Autodesk Inventor part; units mm, degrees
(part 2 of 2)
  arc A261 (1763.513924, 763.538309) -> (1755.513924, 771.538309) centre (1755.513924, 763.538309) ccw
  arc A262 (1755.513924, 731.538309) -> (1763.513924, 739.538309) centre (1755.513924, 739.538309) ccw
  arc A263 (1723.513924, 739.538309) -> (1731.513924, 731.538309) centre (1731.513924, 739.538309) ccw
  line L266 (2481.513924, 771.538309) -> (2505.513924, 771.538309)
  line L267 (2513.513924, 763.538309) -> (2513.513924, 739.538309)
  line L268 (2505.513924, 731.538309) -> (2481.513924, 731.538309)
  line L269 (2473.513924, 739.538309) -> (2473.513924, 763.538309)
  arc A264 (2481.513924, 771.538309) -> (2473.513924, 763.538309) centre (2481.513924, 763.538309) ccw
  arc A265 (2513.513924, 763.538309) -> (2505.513924, 771.538309) centre (2505.513924, 763.538309) ccw
  arc A266 (2505.513924, 731.538309) -> (2513.513924, 739.538309) centre (2505.513924, 739.538309) ccw
  arc A267 (2473.513924, 739.538309) -> (2481.513924, 731.538309) centre (2481.513924, 739.538309) ccw
  line L270 (3231.513924, 771.538309) -> (3255.513924, 771.538309)
  line L271 (3263.513924, 763.538309) -> (3263.513924, 739.538309)
  line L272 (3255.513924, 731.538309) -> (3231.513924, 731.538309)
  line L273 (3223.513924, 739.538309) -> (3223.513924, 763.538309)
  arc A268 (3231.513924, 771.538309) -> (3223.513924, 763.538309) centre (3231.513924, 763.538309) ccw
  arc A269 (3263.513924, 763.538309) -> (3255.513924, 771.538309) centre (3255.513924, 763.538309) ccw
  arc A270 (3255.513924, 731.538309) -> (3263.513924, 739.538309) centre (3255.513924, 739.538309) ccw
  arc A271 (3223.513924, 739.538309) -> (3231.513924, 731.538309) centre (3231.513924, 739.538309) ccw
  line L274 (3981.513924, 771.538309) -> (4005.513924, 771.538309)
  line L275 (4013.513924, 763.538309) -> (4013.513924, 739.538309)
  line L276 (4005.513924, 731.538309) -> (3981.513924, 731.538309)
  line L277 (3973.513924, 739.538309) -> (3973.513924, 763.538309)
  arc A272 (3981.513924, 771.538309) -> (3973.513924, 763.538309) centre (3981.513924, 763.538309) ccw
  arc A273 (4013.513924, 763.538309) -> (4005.513924, 771.538309) centre (4005.513924, 763.538309) ccw
  arc A274 (4005.513924, 731.538309) -> (4013.513924, 739.538309) centre (4005.513924, 739.538309) ccw
  arc A275 (3973.513924, 739.538309) -> (3981.513924, 731.538309) centre (3981.513924, 739.538309) ccw
  line L278 (4731.513924, 771.538309) -> (4755.513924, 771.538309)
  line L279 (4763.513924, 763.538309) -> (4763.513924, 739.538309)
  line L280 (4755.513924, 731.538309) -> (4731.513924, 731.538309)
  line L281 (4723.513924, 739.538309) -> (4723.513924, 763.538309)
  arc A276 (4731.513924, 771.538309) -> (4723.513924, 763.538309) centre (4731.513924, 763.538309) ccw
  arc A277 (4763.513924, 763.538309) -> (4755.513924, 771.538309) centre (4755.513924, 763.538309) ccw
  arc A278 (4755.513924, 731.538309) -> (4763.513924, 739.538309) centre (4755.513924, 739.538309) ccw
  arc A279 (4723.513924, 739.538309) -> (4731.513924, 731.538309) centre (4731.513924, 739.538309) ccw
  line L282 (231.513924, 21.538309) -> (255.513924, 21.538309)
  line L283 (263.513924, 13.538309) -> (263.513924, -10.461691)
  line L284 (255.513924, -18.461691) -> (231.513924, -18.461691)
  line L285 (223.513924, -10.461691) -> (223.513924, 13.538309)
  arc A280 (231.513924, 21.538309) -> (223.513924, 13.538309) centre (231.513924, 13.538309) ccw
  arc A281 (263.513924, 13.538309) -> (255.513924, 21.538309) centre (255.513924, 13.538309) ccw
  arc A282 (255.513924, -18.461691) -> (263.513924, -10.461691) centre (255.513924, -10.461691) ccw
  arc A283 (223.513924, -10.461691) -> (231.513924, -18.461691) centre (231.513924, -10.461691) ccw
  line L286 (981.513924, 21.538309) -> (1005.513924, 21.538309)
  line L287 (1013.513924, 13.538309) -> (1013.513924, -10.461691)
  line L288 (1005.513924, -18.461691) -> (981.513924, -18.461691)
  line L289 (973.513924, -10.461691) -> (973.513924, 13.538309)
  arc A284 (981.513924, 21.538309) -> (973.513924, 13.538309) centre (981.513924, 13.538309) ccw
  arc A285 (1013.513924, 13.538309) -> (1005.513924, 21.538309) centre (1005.513924, 13.538309) ccw
  arc A286 (1005.513924, -18.461691) -> (1013.513924, -10.461691) centre (1005.513924, -10.461691) ccw
  arc A287 (973.513924, -10.461691) -> (981.513924, -18.461691) centre (981.513924, -10.461691) ccw
  line L290 (1731.513924, 21.538309) -> (1755.513924, 21.538309)
  line L291 (1763.513924, 13.538309) -> (1763.513924, -10.461691)
  line L292 (1755.513924, -18.461691) -> (1731.513924, -18.461691)
  line L293 (1723.513924, -10.461691) -> (1723.513924, 13.538309)
  arc A288 (1731.513924, 21.538309) -> (1723.513924, 13.538309) centre (1731.513924, 13.538309) ccw
  arc A289 (1763.513924, 13.538309) -> (1755.513924, 21.538309) centre (1755.513924, 13.538309) ccw
  arc A290 (1755.513924, -18.461691) -> (1763.513924, -10.461691) centre (1755.513924, -10.461691) ccw
  arc A291 (1723.513924, -10.461691) -> (1731.513924, -18.461691) centre (1731.513924, -10.461691) ccw
  line L294 (2481.513924, 21.538309) -> (2505.513924, 21.538309)
  line L295 (2513.513924, 13.538309) -> (2513.513924, -10.461691)
  line L296 (2505.513924, -18.461691) -> (2481.513924, -18.461691)
  line L297 (2473.513924, -10.461691) -> (2473.513924, 13.538309)
  arc A292 (2481.513924, 21.538309) -> (2473.513924, 13.538309) centre (2481.513924, 13.538309) ccw
  arc A293 (2513.513924, 13.538309) -> (2505.513924, 21.538309) centre (2505.513924, 13.538309) ccw
  arc A294 (2505.513924, -18.461691) -> (2513.513924, -10.461691) centre (2505.513924, -10.461691) ccw
  arc A295 (2473.513924, -10.461691) -> (2481.513924, -18.461691) centre (2481.513924, -10.461691) ccw
  line L298 (3231.513924, 21.538309) -> (3255.513924, 21.538309)
  line L299 (3263.513924, 13.538309) -> (3263.513924, -10.461691)
  line L300 (3255.513924, -18.461691) -> (3231.513924, -18.461691)
  line L301 (3223.513924, -10.461691) -> (3223.513924, 13.538309)
  arc A296 (3231.513924, 21.538309) -> (3223.513924, 13.538309) centre (3231.513924, 13.538309) ccw
  arc A297 (3263.513924, 13.538309) -> (3255.513924, 21.538309) centre (3255.513924, 13.538309) ccw
  arc A298 (3255.513924, -18.461691) -> (3263.513924, -10.461691) centre (3255.513924, -10.461691) ccw
  arc A299 (3223.513924, -10.461691) -> (3231.513924, -18.461691) centre (3231.513924, -10.461691) ccw
  line L302 (3981.513924, 21.538309) -> (4005.513924, 21.538309)
  line L303 (4013.513924, 13.538309) -> (4013.513924, -10.461691)
  line L304 (4005.513924, -18.461691) -> (3981.513924, -18.461691)
  line L305 (3973.513924, -10.461691) -> (3973.513924, 13.538309)
  arc A300 (3981.513924, 21.538309) -> (3973.513924, 13.538309) centre (3981.513924, 13.538309) ccw
  arc A301 (4013.513924, 13.538309) -> (4005.513924, 21.538309) centre (4005.513924, 13.538309) ccw
  arc A302 (4005.513924, -18.461691) -> (4013.513924, -10.461691) centre (4005.513924, -10.461691) ccw
  arc A303 (3973.513924, -10.461691) -> (3981.513924, -18.461691) centre (3981.513924, -10.461691) ccw
  line L306 (4731.513924, 21.538309) -> (4755.513924, 21.538309)
  line L307 (4763.513924, 13.538309) -> (4763.513924, -10.461691)
  line L308 (4755.513924, -18.461691) -> (4731.513924, -18.461691)
  line L309 (4723.513924, -10.461691) -> (4723.513924, 13.538309)
  arc A304 (4731.513924, 21.538309) -> (4723.513924, 13.538309) centre (4731.513924, 13.538309) ccw
  arc A305 (4763.513924, 13.538309) -> (4755.513924, 21.538309) centre (4755.513924, 13.538309) ccw
  arc A306 (4755.513924, -18.461691) -> (4763.513924, -10.461691) centre (4755.513924, -10.461691) ccw
  arc A307 (4723.513924, -10.461691) -> (4731.513924, -18.461691) centre (4731.513924, -10.461691) ccw
  point P0 (0, 0)
  point P1 (263.513924, 7481.538309)
  point P2 (263.513924, 7521.538309)
  point P3 (223.513924, 7481.538309)
  point P4 (1013.513924, 7481.538309)
  point P5 (1013.513924, 7521.538309)
  point P6 (973.513924, 7481.538309)
  point P7 (1763.513924, 7481.538309)
  point P8 (1763.513924, 7521.538309)
  point P9 (1723.513924, 7481.538309)
  point P10 (2513.513924, 7481.538309)
  point P11 (2513.513924, 7521.538309)
  point P12 (2473.513924, 7481.538309)
  point P13 (3263.513924, 7481.538309)
  point P14 (3263.513924, 7521.538309)
  point P15 (3223.513924, 7481.538309)
  point P16 (4013.513924, 7481.538309)
  point P17 (4013.513924, 7521.538309)
  point P18 (3973.513924, 7481.538309)
  point P19 (4763.513924, 7481.538309)
  point P20 (4763.513924, 7521.538309)
  point P21 (4723.513924, 7481.538309)
  point P22 (263.513924, 6731.538309)
  point P23 (263.513924, 6771.538309)
  point P24 (223.513924, 6731.538309)
  point P25 (1013.513924, 6731.538309)
  point P26 (1013.513924, 6771.538309)
  point P27 (973.513924, 6731.538309)
  point P28 (1763.513924, 6731.538309)
  point P29 (1763.513924, 6771.538309)
  point P30 (1723.513924, 6731.538309)
  point P31 (2513.513924, 6731.538309)
  point P32 (2513.513924, 6771.538309)
  point P33 (2473.513924, 6731.538309)
  point P34 (3263.513924, 6731.538309)
  point P35 (3263.513924, 6771.538309)
  point P36 (3223.513924, 6731.538309)
  point P37 (4013.513924, 6731.538309)
  point P38 (4013.513924, 6771.538309)
  point P39 (3973.513924, 6731.538309)
  point P40 (4763.513924, 6731.538309)
  point P41 (4763.513924, 6771.538309)
  point P42 (4723.513924, 6731.538309)
  point P43 (263.513924, 5981.538309)
  point P44 (263.513924, 6021.538309)
  point P45 (223.513924, 5981.538309)
  point P46 (1013.513924, 5981.538309)
  point P47 (1013.513924, 6021.538309)
  point P48 (973.513924, 5981.538309)
  point P49 (1763.513924, 5981.538309)
  point P50 (1763.513924, 6021.538309)
  point P51 (1723.513924, 5981.538309)
  point P52 (2513.513924, 5981.538309)
  point P53 (2513.513924, 6021.538309)
  point P54 (2473.513924, 5981.538309)
  point P55 (3263.513924, 5981.538309)
  point P56 (3263.513924, 6021.538309)
  point P57 (3223.513924, 5981.538309)
  point P58 (4013.513924, 5981.538309)
  point P59 (4013.513924, 6021.538309)
  point P60 (3973.513924, 5981.538309)
  point P61 (4763.513924, 5981.538309)
  point P62 (4763.513924, 6021.538309)
  point P63 (4723.513924, 5981.538309)
  point P64 (263.513924, 5231.538309)
  point P65 (263.513924, 5271.538309)
  point P66 (223.513924, 5231.538309)
  point P67 (1013.513924, 5231.538309)
  point P68 (1013.513924, 5271.538309)
  point P69 (973.513924, 5231.538309)
  point P70 (1763.513924, 5231.538309)
  point P71 (1763.513924, 5271.538309)
  point P72 (1723.513924, 5231.538309)
  point P73 (2513.513924, 5231.538309)
  point P74 (2513.513924, 5271.538309)
  point P75 (2473.513924, 5231.538309)
  point P76 (3263.513924, 5231.538309)
  point P77 (3263.513924, 5271.538309)
  point P78 (3223.513924, 5231.538309)
  point P79 (4013.513924, 5231.538309)
  point P80 (4013.513924, 5271.538309)
  point P81 (3973.513924, 5231.538309)
  point P82 (4763.513924, 5231.538309)
  point P83 (4763.513924, 5271.538309)
  point P84 (4723.513924, 5231.538309)
  point P85 (263.513924, 4481.538309)
  point P86 (263.513924, 4521.538309)
  point P87 (223.513924, 4481.538309)
  point P88 (1013.513924, 4481.538309)
  point P89 (1013.513924, 4521.538309)
  point P90 (973.513924, 4481.538309)
  point P91 (1763.513924, 4481.538309)
  point P92 (1763.513924, 4521.538309)
  point P93 (1723.513924, 4481.538309)
  point P94 (2513.513924, 4481.538309)
  point P95 (2513.513924, 4521.538309)
  point P96 (2473.513924, 4481.538309)
  point P97 (3263.513924, 4481.538309)
  point P98 (3263.513924, 4521.538309)
  point P99 (3223.513924, 4481.538309)
  point P100 (4013.513924, 4481.538309)
  point P101 (4013.513924, 4521.538309)
  point P102 (3973.513924, 4481.538309)
  point P103 (4763.513924, 4481.538309)
  point P104 (4763.513924, 4521.538309)
  point P105 (4723.513924, 4481.538309)
  point P106 (263.513924, 3731.538309)
  point P107 (263.513924, 3771.538309)
  point P108 (223.513924, 3731.538309)
  point P109 (1013.513924, 3731.538309)
  point P110 (1013.513924, 3771.538309)
  point P111 (973.513924, 3731.538309)
  point P112 (1763.513924, 3731.538309)
  point P113 (1763.513924, 3771.538309)
  point P114 (1723.513924, 3731.538309)
  point P115 (2513.513924, 3731.538309)
  point P116 (2513.513924, 3771.538309)
  point P117 (2473.513924, 3731.538309)
  point P118 (3263.513924, 3731.538309)
  point P119 (3263.513924, 3771.538309)
  point P120 (3223.513924, 3731.538309)
  point P121 (4013.513924, 3731.538309)
  point P122 (4013.513924, 3771.538309)
  point P123 (3973.513924, 3731.538309)
  point P124 (4763.513924, 3731.538309)
  point P125 (4763.513924, 3771.538309)
  point P126 (4723.513924, 3731.538309)
  point P127 (263.513924, 2981.538309)
  point P128 (263.513924, 3021.538309)
  point P129 (223.513924, 2981.538309)
  point P130 (1013.513924, 2981.538309)
  point P131 (1013.513924, 3021.538309)
  point P132 (973.513924, 2981.538309)
  point P133 (1763.513924, 2981.538309)
  point P134 (1763.513924, 3021.538309)
  point P135 (1723.513924, 2981.538309)
  point P136 (2513.513924, 2981.538309)
  point P137 (2513.513924, 3021.538309)
  point P138 (2473.513924, 2981.538309)
  point P139 (3263.513924, 2981.538309)
  point P140 (3263.513924, 3021.538309)
  point P141 (3223.513924, 2981.538309)
  point P142 (4013.513924, 2981.538309)
  point P143 (4013.513924, 3021.538309)
  point P144 (3973.513924, 2981.538309)
  point P145 (4763.513924, 2981.538309)
  point P146 (4763.513924, 3021.538309)
  point P147 (4723.513924, 2981.538309)
  point P148 (263.513924, 2231.538309)
  point P149 (263.513924, 2271.538309)
  point P150 (223.513924, 2231.538309)
  point P151 (1013.513924, 2231.538309)
  point P152 (1013.513924, 2271.538309)
  point P153 (973.513924, 2231.538309)
  point P154 (1763.513924, 2231.538309)
  point P155 (1763.513924, 2271.538309)
  point P156 (1723.513924, 2231.538309)
  point P157 (2513.513924, 2231.538309)
  point P158 (2513.513924, 2271.538309)
  point P159 (2473.513924, 2231.538309)
  point P160 (3263.513924, 2231.538309)
  point P161 (3263.513924, 2271.538309)
  point P162 (3223.513924, 2231.538309)
  point P163 (4013.513924, 2231.538309)
  point P164 (4013.513924, 2271.538309)
  point P165 (3973.513924, 2231.538309)
  point P166 (4763.513924, 2231.538309)
  point P167 (4763.513924, 2271.538309)
  point P168 (4723.513924, 2231.538309)
  point P169 (263.513924, 1481.538309)
  point P170 (263.513924, 1521.538309)
  point P171 (223.513924, 1481.538309)
  point P172 (1013.513924, 1481.538309)
  point P173 (1013.513924, 1521.538309)
  point P174 (973.513924, 1481.538309)
  point P175 (1763.513924, 1481.538309)
  point P176 (1763.513924, 1521.538309)
  point P177 (1723.513924, 1481.538309)
  point P178 (2513.513924, 1481.538309)
  point P179 (2513.513924, 1521.538309)
  point P180 (2473.513924, 1481.538309)
  point P181 (3263.513924, 1481.538309)
  point P182 (3263.513924, 1521.538309)
  point P183 (3223.513924, 1481.538309)
  point P184 (4013.513924, 1481.538309)
  point P185 (4013.513924, 1521.538309)
  point P186 (3973.513924, 1481.538309)
  point P187 (4763.513924, 1481.538309)
  point P188 (4763.513924, 1521.538309)
  point P189 (4723.513924, 1481.538309)
  point P190 (263.513924, 731.538309)
  point P191 (263.513924, 771.538309)
  point P192 (223.513924, 731.538309)
  point P193 (1013.513924, 731.538309)
  point P194 (1013.513924, 771.538309)
  point P195 (973.513924, 731.538309)
  point P196 (1763.513924, 731.538309)
  point P197 (1763.513924, 771.538309)
  point P198 (1723.513924, 731.538309)
  point P199 (2513.513924, 731.538309)
  dimension "d2" = 40
  dimension "d3" = 40
  dimension "d5" = 40
  dimension "d6" = 8
  dimension "d9" = 750
  dimension "d12" = 750
  dimension "d36" = 40
  constraints: 616 end point, 616 point on circle, 462 point on line, 308 centre point, 8 tangent, 3 equal radius, 2 horizontal, 2 parallel, 1 perpendicular, 1 vertical, 1748 other
  measures "d2" distance of point (263.514, 7481.538) point (223.514, 7481.538)
  measures "d3" distance of point (263.514, 7521.538) point (263.514, 7481.538)
  measures "d5" distance between parallel lines of L5 L3
  measures "d6" radius of A0
  measures "d9" distance of point (263.514, 7481.538) point (1013.514, 7481.538)
  measures "d12" distance of point (263.514, 7481.538) point (263.514, 6731.538)
  measures "d36" distance between parallel lines of L4 L0
extrude "Extrusion2" add sketch "Sketch2" along normal blind 850 contours L0 A1 L1 A2 L2 A3 L3 A0 | L6 A5 L7 A6 L8 A7 L9 A4 | L10 A9 L11 A10 L12 A11 L13 A8 | L14 A13 L15 A14 L16 A15 L17 A12 | L18 A17 L19 A18 L20 A19 L21 A16 | L22 A21 L23 A22 L24 A23 L25 A20 | L26 A25 L27 A26 L28 A27 L29 A24 | L30 A29 L31 A30 L32 A31 L33 A28 | L54 A53 L55 A54 L56 A55 L57 A52 | L58 A57 L59 A58 L60 A59 L61 A56 | L82 A81 L83 A82 L84 A83 L85 A80 | L86 A85 L87 A86 L88 A87 L89 A84 | L110 A109 L111 A110 L112 A111 L113 A108 | L114 A113 L115 A114 L116 A115 L117 A112 | L122 A121 L123 A122 L124 A123 L125 A120 | L126 A125 L127 A126 L128 A127 L129 A124 | L130 A129 L131 A130 L132 A131 L133 A128 | L138 A137 L139 A138 L140 A139 L141 A136 | L142 A141 L143 A142 L144 A143 L145 A140 | L150 A149 L151 A150 L152 A151 L153 A148 | L158 A157 L159 A158 L160 A159 L161 A156 | L166 A165 L167 A166 L168 A167 L169 A164 | L170 A169 L171 A170 L172 A171 L173 A168 | L178 A177 L179 A178 L180 A179 L181 A176 | L182 A181 L183 A182 L184 A183 L185 A180 | L186 A185 L187 A186 L188 A187 L189 A184 | L194 A193 L195 A194 L196 A195 L197 A192 | L198 A197 L199 A198 L200 A199 L201 A196 | L222 A221 L223 A222 L224 A223 L225 A220 | L226 A225 L227 A226 L228 A227 L229 A224 | L250 A249 L251 A250 L252 A251 L253 A248 | L254 A253 L255 A254 L256 A255 L257 A252 | L278 A277 L279 A278 L280 A279 L281 A276 | L282 A281 L283 A282 L284 A283 L285 A280 | L286 A285 L287 A286 L288 A287 L289 A284 | L290 A289 L291 A290 L292 A291 L293 A288 | L294 A293 L295 A294 L296 A295 L297 A292 | L298 A297 L299 A298 L300 A299 L301 A296 | L302 A301 L303 A302 L304 A303 L305 A300 | L306 A305 L307 A306 L308 A307 L309 A304
sketch "Sketch3" plane through (0, 0, 870) normal (0, 0, 1) x (1, 0, 0)
  line L0 (223.513924, -18.461691) -> (4763.513924, -18.461691)
  line L1 (4763.513924, -18.461691) -> (4763.513924, 21.538309)
  line L2 (4763.513924, 21.538309) -> (223.513924, 21.538309)
  line L3 (223.513924, 21.538309) -> (223.513924, -18.461691)
  arc A0 (223.513924, -10.461691) -> (231.513924, -18.461691) centre (231.513924, -10.461691) ccw
  line L4 (223.513924, -10.461691) -> (223.513924, -18.461691) construction
  line L5 (223.513924, -18.461691) -> (231.513924, -18.461691) construction
  line L6 (4763.513924, -18.461691) -> (4723.513924, -18.461691)
  line L7 (4723.513924, -18.461691) -> (4723.513924, 7521.538309)
  line L8 (4723.513924, 7521.538309) -> (4763.513924, 7521.538309)
  line L9 (4763.513924, 7521.538309) -> (4763.513924, -18.461691)
  line L10 (4763.513924, 7521.538309) -> (223.513924, 7521.538309)
  line L11 (223.513924, 7521.538309) -> (223.513924, 7481.538309)
  line L12 (223.513924, 7481.538309) -> (4763.513924, 7481.538309)
  line L13 (4763.513924, 7481.538309) -> (4763.513924, 7521.538309)
  line L14 (223.513924, 7521.538309) -> (263.513924, 7521.538309)
  line L15 (263.513924, 7521.538309) -> (263.513924, -18.461691)
  line L16 (263.513924, -18.461691) -> (223.513924, -18.461691)
  line L17 (223.513924, -18.461691) -> (223.513924, 7521.538309)
  point P0 (0, 0)
  point P1 (4723.513924, 21.538309)
  point P2 (263.513924, 21.538309)
  point P3 (263.513924, 7481.538309)
  point P4 (4723.513924, 7481.538309)
  dimension "d17" = 4540
  dimension "d18" = 40
  dimension "d19" = 40
  dimension "d20" = 7540
  dimension "d21" = 4540
  dimension "d22" = 40
  dimension "d23" = 40
  constraints: 36 end point, 8 parallel, 5 horizontal, 4 perpendicular, 1 point on line, 1 vertical
  measures "d17" distance of L2.end L1.end
  measures "d18" distance of L1.end L0.end
  measures "d19" distance of L7.end L8.end
  measures "d20" distance of L6.end L7.end
  measures "d21" distance of L12.end L11.end
  measures "d22" distance of L11.end L10.end
  measures "d23" distance between parallel lines of L17 L15
extrude "Extrusion3" add sketch "Sketch3" along normal blind 40 contours L3 A0 L0 | A0 L3 L2 L15 L0 | L15 L2 L7 L0 | L17 L12 L15 L2 | L7 L2 L1 L0 | L11 L10 L15 L12 | L7 L12 L9 L2 | L15 L10 L7 L12 | L7 L8 L9 L12
sketch "Sketch4" plane through (0, 0, 870) normal (0, 0, 1) x (1, 0, 0)
  line L0 (1723.513924, 4521.538309) -> (3263.513924, 4521.538309)
  line L1 (3263.513924, 4521.538309) -> (3263.513924, 4481.538309)
  line L2 (3263.513924, 4481.538309) -> (1723.513924, 4481.538309)
  line L3 (1723.513924, 4481.538309) -> (1723.513924, 4521.538309)
  line L4 (1731.513924, 4521.538309) -> (1723.513924, 4521.538309) construction
  arc A0 (1731.513924, 4521.538309) -> (1723.513924, 4513.538309) centre (1731.513924, 4513.538309) ccw construction
  line L5 (1723.513924, 4521.538309) -> (1723.513924, 4513.538309) construction
  line L6 (3263.513924, 4521.538309) -> (3223.513924, 4521.538309)
  line L7 (3223.513924, 4521.538309) -> (3223.513924, 2981.538309)
  line L8 (3223.513924, 2981.538309) -> (3263.513924, 2981.538309)
  line L9 (3263.513924, 2981.538309) -> (3263.513924, 4521.538309)
  line L10 (3263.513924, 2981.538309) -> (1723.513924, 2981.538309)
  line L11 (1723.513924, 2981.538309) -> (1723.513924, 3021.538309)
  line L12 (1723.513924, 3021.538309) -> (3263.513924, 3021.538309)
  line L13 (3263.513924, 3021.538309) -> (3263.513924, 2981.538309)
  line L14 (1723.513924, 2981.538309) -> (1763.513924, 2981.538309)
  line L15 (1763.513924, 2981.538309) -> (1763.513924, 4521.538309)
  line L16 (1763.513924, 4521.538309) -> (1723.513924, 4521.538309)
  line L17 (1723.513924, 4521.538309) -> (1723.513924, 2981.538309)
  point P0 (0, 0)
  point P1 (3223.513924, 4481.538309)
  point P2 (3223.513924, 3021.538309)
  point P3 (1763.513924, 3021.538309)
  point P4 (1763.513924, 4481.538309)
  dimension "d26" = 1540
  dimension "d27" = 40
  dimension "d28" = 40
  dimension "d29" = 1540
  dimension "d30" = 1540
  dimension "d31" = 40
  dimension "d32" = 40
  dimension "d33" = 1540
  constraints: 36 end point, 8 parallel, 5 horizontal, 4 perpendicular, 1 vertical
  measures "d26" distance of L1.end L2.end
  measures "d27" distance of L0.end L1.end
  measures "d28" distance of L8.end L7.end
  measures "d29" distance of L7.end L6.end
  measures "d30" distance of L11.end L12.end
  measures "d31" distance of L10.end L11.end
  measures "d32" distance of L16.end L15.end
  measures "d33" distance of L15.end L14.end
extrude "Extrusion4" add sketch "Sketch4" along normal blind 40 contours L0 L15 L2 L3 | L0 L7 L2 L15 | L2 L15 L12 L17 | L0 L1 L2 L7 | L12 L15 L10 L11 | L2 L9 L12 L7 | L12 L7 L10 L15 | L12 L9 L8 L7
body "Solid1"
